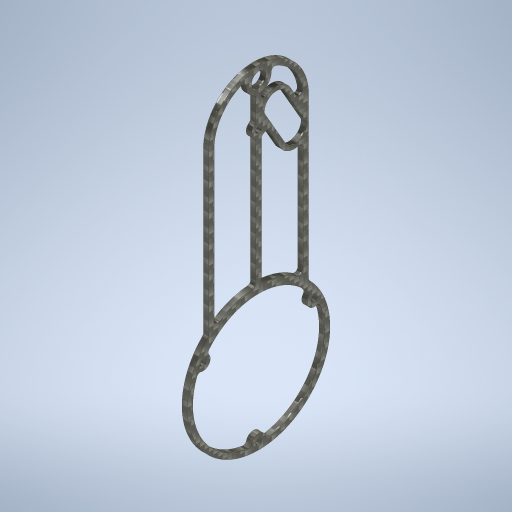
# Autodesk Inventor part: LowerArmFrame
Saved by Autodesk Inventor 2024.2 (Build 282272000, 272)
## iProperties
Created: 2024-01-18
Part Number: LowerArmFrame
Material: CFRP
Document SubType Name: Modeling
Designer: Masato Kubotera
Density: 1.43 g/cm^3
Appearance: Carbon Fiber 1
Mass: 12.7324 g
Surface Area: 100.038 cm^2
Volume: 8.90374 cm^3
Vendor: ALLPCB
Author: Masato Kubotera
Autodesk Inventor part; units mm, degrees
ref_plane "YZ Plane" through (0, 0, 0) normal (1, 0, 0) x (0, 1, 0)
ref_plane "XZ Plane" through (0, 0, 0) normal (0, 1, 0) x (-1, 0, 0)
ref_plane "XY Plane" through (0, 0, 0) normal (0, 0, 1) x (1, 0, 0)
sketch "Sketch1" plane through (0, 0, 0) normal (0, 1, 0) x (-1, 0, 0)
  line L0 (-28, -21) -> (-28, -110.6061)
  line L1 (0, 0) -> (0, -180) construction
  arc A0 (-28.5714, -112.0058) -> (28.5714, -112.0058) centre (0, -140) ccw
  line L2 (28, -21) -> (28, -110.6061)
  circle A1 centre (0, 0) radius 4 construction
  line L3 (0, 0) -> (20, -34.641) construction
  circle A2 centre (10, -17.3205) radius 20 construction
  circle A3 centre (0, 0) radius 40 construction
  arc A4 (17.3769, -38.8977) -> (24.9979, -34.4977) centre (20, -34.641) ccw construction
  arc A5 (15.9891, -40.194) -> (26.8144, -33.944) centre (20, -34.641) ccw
  line L4 (17.3769, -38.8977) -> (5.0021, -17.4638) construction
  line L5 (15.9891, -40.194) -> (3.1856, -18.0175)
  line L6 (24.9979, -34.4977) -> (12.6231, -13.0638) construction
  line L7 (26.8144, -33.944) -> (14.0109, -11.7675)
  line L8 (11.1895, -28.1808) -> (18.8105, -23.7808) construction
  arc A6 (12.6231, -13.0638) -> (5.0021, -17.4638) centre (10, -17.3205) ccw construction
  arc A7 (14.0109, -11.7675) -> (3.1856, -18.0175) centre (10, -17.3205) ccw
  line L9 (0, 0) -> (20, 0) construction
  line L10 (20, 0) -> (40, 0) construction
  circle A8 centre (0, -140) radius 36 construction
  line L11 (0, -140) -> (-34.641, -120) construction
  line L12 (0, -140) -> (34.641, -120) construction
  arc A9 (28, -21) -> (-28, -21) centre (0, -21) ccw
  line L13 (-25, -104.8574) -> (-25, -21)
  line L14 (-1.5, -29.3734) -> (-1.5, -98.1461)
  arc A10 (-3.3333, -100.1391) -> (-21.9048, -106.5309) centre (0, -140) ccw
  line L15 (25, -104.8574) -> (25, -45.224)
  line L16 (1.5, -29.3734) -> (1.5, -98.1461)
  arc A11 (21.9048, -106.5309) -> (3.3333, -100.1391) centre (0, -140) ccw
  arc A12 (12.2058, -39.141) -> (22.4545, -43.2998) centre (20, -34.641) ccw
  line L17 (12.2058, -39.141) -> (5.7488, -27.9571)
  arc A13 (-9.7809, 2.0072) -> (-25, -21) centre (0, -21) ccw
  arc A14 (-6.9988, 0.1296) -> (-2.7222, -6.449) centre (0, 0) ccw
  arc A15 (17.7942, -12.8205) -> (4.6818, -10.0599) centre (10, -17.3205) ccw
  arc A16 (2.7222, -6.449) -> (6.9988, 0.1296) centre (0, 0) ccw
  arc A17 (24.6789, -17.006) -> (9.7809, 2.0072) centre (0, -21) ccw
  line L18 (20.9725, -18.3255) -> (17.7942, -12.8205)
  circle A18 centre (0, -24.5) radius 4 construction
  arc A19 (-25, -104.8574) -> (-21.9048, -106.5309) centre (-23, -104.8574) ccw
  arc A20 (-3.3333, -100.1391) -> (-1.5, -98.1461) centre (-3.5, -98.1461) ccw
  arc A21 (-1.5, -8.2916) -> (-2.7222, -6.449) centre (-3.5, -8.2916) ccw
  arc A22 (-6.9988, 0.1296) -> (-9.7809, 2.0072) centre (-8.9985, 0.1667) ccw
  arc A23 (9.7809, 2.0072) -> (6.9988, 0.1296) centre (8.9985, 0.1667) ccw
  arc A24 (20.9725, -18.3255) -> (24.6789, -17.006) centre (22.7046, -17.3255) ccw
  arc A25 (5.7488, -27.9571) -> (2.6778, -27.4714) centre (4.0167, -28.9571) ccw
  arc A26 (1.5, -98.1461) -> (3.3333, -100.1391) centre (3.5, -98.1461) ccw
  arc A27 (21.9048, -106.5309) -> (25, -104.8574) centre (23, -104.8574) ccw
  arc A28 (25, -45.224) -> (22.4545, -43.2998) centre (23, -45.224) ccw
  arc A29 (-2.3333, -21.2511) -> (-2.3333, -27.7489) centre (0, -24.5) ccw
  line L19 (-1.5, -8.2916) -> (-1.5, -19.6266)
  arc A30 (-1.5, -29.3734) -> (-2.3333, -27.7489) centre (-3.5, -29.3734) ccw
  arc A31 (-2.3333, -21.2511) -> (-1.5, -19.6266) centre (-3.5, -19.6266) ccw
  arc A32 (-33.823, -124.9997) -> (-28.9876, -118.6524) centre (-31.1769, -122) ccw
  arc A33 (3.9209, -176.7917) -> (-3.9209, -176.7917) centre (0, -176) ccw
  arc A34 (-33.823, -124.9997) -> (-3.9209, -176.7917) centre (0, -140) ccw
  arc A35 (28.9876, -118.6524) -> (33.823, -124.9997) centre (31.1769, -122) ccw
  arc A36 (3.9209, -176.7917) -> (33.823, -124.9997) centre (0, -140) ccw
  arc A37 (28.9876, -118.6524) -> (-28.9876, -118.6524) centre (0, -140) ccw
  arc A38 (-28.5714, -112.0058) -> (-28, -110.6061) centre (-30, -110.6061) ccw
  arc A39 (28, -110.6061) -> (28.5714, -112.0058) centre (30, -110.6061) ccw
  line L20 (1.5, -8.2916) -> (1.5, -8.4464)
  arc A40 (2.7222, -6.449) -> (1.5, -8.2916) centre (3.5, -8.2916) ccw
  arc A41 (1.5, -8.4464) -> (4.6818, -10.0599) centre (3.5, -8.4464) ccw
  arc A42 (2.3333, -27.7489) -> (2.6778, -27.4714) centre (0, -24.5) ccw
  arc A43 (2.3333, -27.7489) -> (1.5, -29.3734) centre (3.5, -29.3734) ccw
  point P0 (-28, -111.4343)
  point P1 (28, -111.4343)
  point P2 (30, -113.5425)
  point P3 (15.9891, -40.194)
  point P4 (-14.0109, -11.7675)
  point P5 (31.1769, -122)
  point P6 (0, 7)
  point P7 (-25, -108.775)
  point P8 (-1.5, -100.0281)
  point P9 (25, -108.775)
  point P10 (1.5, -100.0281)
  point P11 (25, -42.1243)
  point P12 (-2, -6.7082)
  point P13 (25.7858, -19.6697)
  point P14 (-1.5, -20.7919)
  point P15 (-1.5, -28.2081)
  point P16 (-27.7128, -124)
  point P17 (27.7128, -124)
  point P18 (1.5713, -7.7625)
  point P19 (2.2417, -27.8188)
  dimension "d1" = 180
  dimension "d2" = 80
  dimension "d3" = 8
  dimension "d15" = 8.8
  dimension "d16" = 12.5
  dimension "d17" = 10
  dimension "d18" = 1.85
  dimension "d19" = 1.85
  dimension "d20" = 60
  dimension "d21" = 20
  dimension "d22" = 20
  dimension "d24" = 20
  dimension "d29" = 30
  dimension "d31" = 72
  dimension "d32" = 120
  dimension "d40" = 7
  dimension "d41" = 56
  dimension "d43" = 24.5
  dimension "d44" = 3
  dimension "d46" = 3
  dimension "d50" = 8
  dimension "d52" = 2
  dimension "d54" = 3
  dimension "d57" = 9
  dimension "d58" = 8
  constraints: 107 point on circle, 44 centre point, 44 end point, 34 tangent, 22 symmetric about line, 20 coincident, 18 equal radius, 17 point on line, 5 vertical, 3 midpoint, 3 parallel, 2 collinear, 12 other
  measures "d1" distance of L1.start L1.end
  measures "d2" diameter of A0
  measures "d3" diameter of A1
  measures "d15" distance between parallel lines of L6 L4
  measures "d16" distance between parallel lines of L5 L7
  measures "d17" diameter of A4
  measures "d18" distance between parallel lines of L7 L6
  measures "d19" radial gap between concentric circles of A5 A4
  measures "d20" angle of L3 L9
  measures "d21" distance of L9.end L10.end
  measures "d22" radius of A2
  measures "d24" distance of L3.end A6.centre
  measures "d29" angle of L3 L1
  measures "d31" diameter of A8
  measures "d32" angle of L1 L11
  measures "d40" distance of point (0, 7) L3.start
  measures "d41" distance between parallel lines of L0 L2
  measures "d43" distance of point (0, -24.5) point (0, 0)
  measures "d44" distance between parallel lines of L0 L13
  measures "d46" distance between parallel lines of L16 L14
  measures "d50" diameter of A18
  measures "d52" radius of A19
  measures "d54" radial gap between concentric circles of A0 A34
  measures "d57" radius of A12
  measures "d58" diameter of A32
extrude "Extrusion1" add sketch "Sketch1" along normal blind 3
hole "Phi8.0-H7" at (0, 0, 0) direction (0, 1, 0) diameter 8 end through all
hole "Phi3.5" at (31.1769, 0, -122) at (-31.1769, 0, -122) at (0, 0, -176) at (0, 0, -24.5) direction (0, 1, 0) diameter 3.5 end through all
fillet "R2" radius 2 10 edges at (-3.1856, 1.5, -18.0175) (-14.0109, 1.5, -11.7675) (-26.8144, 1.5, -33.944) (-15.9891, 1.5, -40.194) (33.823, 1.5, -124.9997) (-33.823, 1.5, -124.9997) (-3.9209, 1.5, -176.7917) (3.9209, 1.5, -176.7917) (28.9876, 1.5, -118.6524) (-28.9876, 1.5, -118.6524)
equation "\"d19\" = d18"
equation "\"d24\" = d21"
equation "\"d13\" = d5"
equation "\"d5\" = 8.1"
body "Solid1"
